Autodesk Inventor part; units mm, degrees
note: some values were not read from the file. Chosen so that the rebuilt part matches the saved one: direction of "Hole2".
(part 13 of 18)
sketch "Sketch13" plane through (0, 0, 0) normal (1, 0, 0) x (0, 1, 0)
  line L0 (0, -156.7871) -> (0, 91.8442)
  line L1 (0, 25) -> (0, -118.9769)
  line L2 (13.762, 0) -> (-13.762, 0)
  line L3 (-13.762, -20) -> (-13.762, 0)
  line L4 (-0.0006, -82.7054) -> (-0.0006, -41.7054)
  line L5 (6.5385, -24.5854) -> (6.5631, -24.5804)
  ellipse E0 centre (6.6616, -24.5626) end of major axis (7.4453, -24.4021) minor radius 0.0024 (6.8181, -24.5282) -> (6.5631, -24.5804) ccw
  ellipse E1 centre (6.6616, -24.5626) end of major axis (7.4453, -24.4021) minor radius 0.0024 (7.4453, -24.4021) -> (6.9932, -24.4925) ccw
  line L6 (7.4454, -24.4027) -> (7.4453, -24.4021)
  ellipse E2 centre (-6.6543, -24.5616) end of major axis (-7.438, -24.4009) minor radius 0.0024 (-6.9873, -24.4911) -> (-7.438, -24.4009) ccw
  line L7 (-5.6413, -24.7664) -> (-5.4089, -24.8139)
  line L8 (-7.4382, -24.4016) -> (-7.438, -24.4009)
  ellipse E3 centre (6.1292, -24.7063) end of major axis (6.8873, -24.4508) minor radius 0.0023 (6.1976, -24.6808) -> (6.0462, -24.7319) ccw
  ellipse E4 centre (6.1292, -24.7063) end of major axis (6.8873, -24.4508) minor radius 0.0023 (6.3158, -24.6411) -> (6.2034, -24.6789) ccw
  ellipse E5 centre (6.1292, -24.7063) end of major axis (6.8873, -24.4508) minor radius 0.0023 (6.8873, -24.4508) -> (6.7158, -24.5071) ccw
  line L9 (6.89, -24.4589) -> (6.8873, -24.4508)
  line L10 (4.3307, -24.5603) -> (2.6776, -19.6543)
  ellipse E6 centre (8.7715, -25.6199) end of major axis (7.994, -25.8086) minor radius 0.1369 (8.4767, -25.559) -> (8.4597, -25.5643) ccw
  line L11 (8.1889, -25.6311) -> (8.3795, -25.5808)
  ellipse E7 centre (9.0039, -26.5774) end of major axis (8.518, -26.6953) minor radius 0.0856 (8.8835, -26.5204) -> (8.737, -26.7137) ccw
  ellipse E8 centre (-9.6869, -24.5347) end of major axis (-10.4866, -24.5548) minor radius 0.1339 (-10.0381, -24.4229) -> (-10.4866, -24.5548) ccw
  line L12 (-9.714, -24.4015) -> (-8.1405, -24.3541)
  line L13 (-8.1405, -24.3541) -> (-8.1355, -24.5515)
  ellipse E9 centre (-9.6374, -26.5059) end of major axis (-10.4371, -26.526) minor radius 0.1339 (-9.3653, -26.3732) -> (-9.6644, -26.3726) ccw
  line L14 (-8.1405, -24.3541) -> (-8.1504, -23.9607)
  line L15 (-8.1673, -23.2858) -> (-8.1916, -22.3201)
  ellipse E10 centre (-10.031, -10.8352) end of major axis (-12.1204, -10.8877) minor radius 0.3499 (-10.885, -10.5366) -> (-11.1398, -10.5656) ccw
  ellipse E11 centre (-10.0087, -11.7222) end of major axis (-12.0981, -11.7747) minor radius 0.3499 (-10.8714, -11.4245) -> (-11.107, -11.4513) ccw
  ellipse E12 centre (-10.0087, -11.7222) end of major axis (-11.5083, -11.7599) minor radius 0.2511 (-9.2151, -11.4897) -> (-11.4645, -11.818) ccw
  ellipse E13 centre (-9.6374, -26.5059) end of major axis (-10.1372, -26.5184) minor radius 0.0837 (-9.7111, -26.4249) -> (-9.8858, -26.5846) ccw
  ellipse E14 centre (-7.235, -24.4816) end of major axis (-8.033, -24.4244) minor radius 0.0023 (-7.3492, -24.4711) -> (-8.033, -24.4244) ccw
  line L16 (-7.3492, -24.4711) -> (-7.2905, -24.4753)
  line L17 (-7.0539, -24.4922) -> (-5.7945, -24.5819)
  line L18 (-5.7945, -24.5819) -> (-5.8098, -24.7955)
  line L19 (-8.0339, -24.4376) -> (-8.033, -24.4244)
  line L20 (-5.7945, -24.5819) -> (-5.6751, -22.9169)
  line L21 (6.125, -24.1477) -> (6.1927, -24.4898)
  line L22 (5.1567, -24.9711) -> (6.63, -24.6998)
  ellipse E15 centre (6.6974, -24.5888) end of major axis (7.4822, -24.4335) minor radius 0.0964 (6.63, -24.6998) -> (7.3393, -24.4071) ccw
  line L23 (7.3393, -24.4071) -> (6.8175, -24.416)
  line L24 (7.4837, -24.4412) -> (7.4822, -24.4335)
  line L25 (8.6391, -24.2658) -> (8.65, -24.3696)
  line L26 (8.1334, -24.5735) -> (9.0091, -24.4769)
  ellipse E16 centre (9.1156, -24.4999) end of major axis (9.9112, -24.4166) minor radius 0.0342 (9.8759, -24.4103) -> (9.0091, -24.4769) ccw
  ellipse E17 centre (7.6703, -10.688) end of major axis (9.7489, -10.4705) minor radius 0.0893 (9.6066, -10.4531) -> (9.1054, -10.4731) ccw
  ellipse E18 centre (7.7639, -11.5823) end of major axis (9.8425, -11.3648) minor radius 0.0893 (9.6975, -11.3474) -> (9.6301, -11.3478) ccw
  ellipse E19 centre (9.3235, -26.4872) end of major axis (8.8262, -26.5392) minor radius 0.0214 (8.9471, -26.5125) -> (8.8496, -26.5302) ccw
  ellipse E20 centre (9.3235, -26.4872) end of major axis (9.8208, -26.4352) minor radius 0.0214 (9.7809, -26.431) -> (9.5114, -26.4477) ccw
  ellipse E21 centre (-3.2965, -25.8221) end of major axis (-2.5903, -25.9681) minor radius 0.4312 (-4.0047, -25.7714) -> (-3.988, -25.8345) ccw
  line L27 (-7.6925, -23.8764) -> (-7.7511, -24.4362)
  ellipse E22 centre (-9.1083, -24.4985) end of major axis (-8.3127, -24.5819) minor radius 0.0342 (-9.1389, -24.461) -> (-9.8417, -24.4085) ccw
  line L28 (-9.1389, -24.461) -> (-8.1258, -24.5652)
  line L29 (-7.5559, -24.4522) -> (-7.4967, -23.887)
  ellipse E23 centre (-7.6609, -10.6868) end of major axis (-9.7396, -10.469) minor radius 0.0893 (-9.096, -10.4717) -> (-9.5972, -10.4516) ccw
  ellipse E24 centre (-7.7547, -11.5811) end of major axis (-9.8333, -11.3633) minor radius 0.0893 (-9.6209, -11.3463) -> (-9.6883, -11.3459) ccw
  ellipse E25 centre (-7.7547, -11.5811) end of major axis (-9.2465, -11.4248) minor radius 0.0641 (-9.2062, -11.4144) -> (-9.2096, -11.4432) ccw
  ellipse E26 centre (-9.3166, -26.4858) end of major axis (-8.8193, -26.5379) minor radius 0.0214 (-8.8502, -26.542) -> (-8.9401, -26.5111) ccw
  ellipse E27 centre (-9.3166, -26.4858) end of major axis (-9.8139, -26.4337) minor radius 0.0214 (-9.5044, -26.4462) -> (-9.7826, -26.4445) ccw
  line L30 (-4.8207, -21.8442) -> (-5.4206, -24.8731)
  line L31 (-7.1249, -24.4201) -> (-7.2028, -24.4133)
  ellipse E28 centre (-6.6902, -24.5878) end of major axis (-7.4749, -24.4323) minor radius 0.0964 (-7.2028, -24.4133) -> (-6.8152, -24.6604) ccw
  line L32 (-6.8152, -24.6604) -> (-5.2896, -24.9888)
  line L33 (-5.2896, -24.9888) -> (-5.2988, -25.0352)
  line L34 (-7.4764, -24.4401) -> (-7.4749, -24.4323)
  line L35 (-5.345, -24.9535) -> (-5.2896, -24.9888)
  line L36 (-5.2896, -24.9888) -> (-4.6702, -21.8618)
  line L37 (6.9927, -24.4983) -> (7.1608, -24.4862)
  ellipse E29 centre (7.2423, -24.4827) end of major axis (8.0402, -24.4257) minor radius 0.0023 (8.0402, -24.4257) -> (7.1608, -24.4862) ccw
  line L38 (8.0412, -24.4388) -> (8.0402, -24.4257)
  line L39 (5.3972, -21.7895) -> (5.3965, -21.7786)
  line L40 (9.2707, -24.1962) -> (9.2658, -24.3887)
  line L41 (8.0528, -24.399) -> (9.5835, -24.4008)
  ellipse E30 centre (9.6941, -24.5362) end of major axis (10.4939, -24.5564) minor radius 0.1339 (10.4939, -24.5564) -> (9.5835, -24.4008) ccw
  ellipse E31 centre (10.0403, -10.8367) end of major axis (7.951, -10.7839) minor radius 0.3499 (11.1492, -10.5673) -> (10.8944, -10.5383) ccw
  ellipse E32 centre (10.0179, -11.7237) end of major axis (7.9286, -11.6709) minor radius 0.3499 (11.1162, -11.453) -> (10.8807, -11.4262) ccw
  ellipse E33 centre (10.0179, -11.7237) end of major axis (11.5174, -11.7616) minor radius 0.2511 (11.4536, -11.8315) -> (9.2243, -11.4911) ccw
  ellipse E34 centre (9.6692, -25.5218) end of major axis (8.8695, -25.5015) minor radius 0.1339 (9.5586, -25.3864) -> (9.5386, -25.3864) ccw
  ellipse E35 centre (9.6443, -26.5073) end of major axis (9.1445, -26.4947) minor radius 0.0837 (9.8928, -26.5861) -> (9.9159, -26.5843) ccw
  ellipse E36 centre (9.6443, -26.5073) end of major axis (10.1441, -26.52) minor radius 0.0837 (9.9692, -26.4517) -> (9.718, -26.4263) ccw
  line L42 (-8.2953, -25.5869) -> (-8.181, -25.6135)
  ellipse E37 centre (-8.7644, -25.6186) end of major axis (-9.5418, -25.4298) minor radius 0.1369 (-8.4526, -25.563) -> (-8.4712, -25.5572) ccw
  ellipse E38 centre (-8.9969, -26.576) end of major axis (-8.5111, -26.694) minor radius 0.0856 (-8.73, -26.7124) -> (-8.8766, -26.5191) ccw
  ellipse E39 centre (-6.122, -24.7054) end of major axis (-6.8801, -24.4498) minor radius 0.0023 (-6.7099, -24.5056) -> (-6.8801, -24.4498) ccw
  line L43 (-4.9025, -25.6565) -> (-5.0575, -26.1165)
  line L44 (-6.8828, -24.4579) -> (-6.8801, -24.4498)
  line L45 (-3.9973, -22.9715) -> (-2.7633, -19.311)
  line L46 (-4.8183, -25.9908) -> (-5.0575, -26.1165)
  line L47 (-5.0575, -26.1165) -> (-5.0809, -26.1089)
  line L48 (-5.3806, -26.0077) -> (-5.0575, -26.1165)
  line L49 (6.358, -24.6267) -> (6.5138, -24.5921)
  ellipse E40 centre (6.5935, -24.5771) end of major axis (7.3746, -24.4044) minor radius 0.0026 (6.6422, -24.5638) -> (6.5138, -24.5921) ccw
  ellipse E41 centre (6.5935, -24.5771) end of major axis (7.3746, -24.4044) minor radius 0.0026 (6.7584, -24.5381) -> (6.6452, -24.5631) ccw
  ellipse E42 centre (6.5935, -24.5771) end of major axis (7.3746, -24.4044) minor radius 0.0026 (7.3746, -24.4044) -> (6.9573, -24.4944) ccw
  line L50 (7.3751, -24.4065) -> (7.3746, -24.4044)
  ellipse E43 centre (9.3228, -26.6242) end of major axis (10.1179, -26.5359) minor radius 0.2631 (8.6364, -26.8259) -> (8.7826, -26.8719) ccw
  ellipse E44 centre (9.3228, -26.6242) end of major axis (10.1179, -26.5359) minor radius 0.2631 (9.8842, -26.7562) -> (10.0487, -26.6608) ccw
  ellipse E45 centre (-9.3159, -26.6228) end of major axis (-10.111, -26.5344) minor radius 0.2631 (-9.8452, -26.3729) -> (-9.9962, -26.4182) ccw
  ellipse E46 centre (-9.3159, -26.6228) end of major axis (-10.111, -26.5344) minor radius 0.2631 (-10.0265, -26.4334) -> (-10.0354, -26.4386) ccw
  ellipse E47 centre (-9.3159, -26.6228) end of major axis (-10.111, -26.5344) minor radius 0.2631 (-10.102, -26.5857) -> (-9.8773, -26.7547) ccw
  ellipse E48 centre (-9.3159, -26.6228) end of major axis (-8.5208, -26.7113) minor radius 0.2631 (-8.7757, -26.8706) -> (-8.6295, -26.8246) ccw
  line L51 (4.4092, -25.3666) -> (4.5281, -25.3204)
  ellipse E49 centre (5.9388, -24.7753) end of major axis (6.6846, -24.4859) minor radius 0.0025 (6.0605, -24.7254) -> (6.044, -24.7318) ccw
  ellipse E50 centre (5.9388, -24.7753) end of major axis (6.6846, -24.4859) minor radius 0.0025 (6.1548, -24.6889) -> (6.1064, -24.7077) ccw
  ellipse E51 centre (5.9388, -24.7753) end of major axis (6.6846, -24.4859) minor radius 0.0025 (6.6846, -24.4859) -> (6.6131, -24.5125) ccw
  line L52 (4.7709, -26.2989) -> (4.4092, -25.3666)
  ellipse E52 centre (6.6622, -26.6398) end of major axis (5.9164, -26.9292) minor radius 0.0025 (6.3614, -26.7541) -> (6.3717, -26.755) ccw
  line L53 (5.9164, -26.9292) -> (5.5547, -25.9969)
  line L54 (6.6905, -24.5011) -> (6.6846, -24.4859)
  line L55 (4.4092, -25.3666) -> (2.4772, -20.3874)
  line L56 (5.5556, -25.9992) -> (4.7709, -26.2989)
  line L57 (4.7709, -26.2989) -> (4.4206, -26.1135)
  ellipse E53 centre (4.7483, -25.9883) end of major axis (3.8736, -25.6036) minor radius 0.2554 (3.8766, -25.6768) -> (4.4206, -26.1135) ccw
  line L58 (3.8766, -25.6768) -> (2.3761, -21.8095)
  ellipse E54 centre (6.3005, -25.7075) end of major axis (5.5547, -25.9969) minor radius 0.0025 (5.7011, -25.9386) -> (5.5547, -25.9969) ccw
  line L59 (4.7709, -26.2989) -> (5.6964, -25.9395)
  ellipse E55 centre (6.6622, -26.6398) end of major axis (6.1961, -26.8207) minor radius 0.0015 (6.3638, -26.7544) -> (6.3692, -26.7548) ccw
  ellipse E56 centre (8.6322, -25.6643) end of major axis (7.8635, -25.8859) minor radius 0.1461 (8.4225, -25.5765) -> (8.1906, -25.6627) ccw
  line L60 (8.1897, -25.6455) -> (8.4148, -25.5772)
  ellipse E57 centre (8.9045, -26.609) end of major axis (8.4241, -26.7475) minor radius 0.0913 (8.8813, -26.5207) -> (8.7454, -26.7428) ccw
  ellipse E58 centre (8.9045, -26.609) end of major axis (8.1358, -26.8306) minor radius 0.1461 (8.5773, -26.5625) -> (8.6364, -26.8259) ccw
  line L61 (8.1358, -26.8306) -> (8.0248, -26.4453)
  line L62 (0.6093, -23.6195) -> (0.581, -23.1628)
  line L63 (-4.4761, -26.0441) -> (-4.3988, -26.1802)
  line L64 (-4.3988, -26.1802) -> (-3.922, -26.0734)
  ellipse E59 centre (-2.6442, -26.5919) end of major axis (-3.4175, -26.7969) minor radius 0.1421 (-3.4175, -26.7969) -> (-2.9999, -26.8134) ccw
  line L65 (-3.4175, -26.7969) -> (-3.5926, -26.1367)
  line L66 (-9.1967, -24.375) -> (-9.2054, -24.2017)
  line L67 (-8.4493, -24.2774) -> (-8.4463, -24.3379)
  ellipse E60 centre (-9.7984, -24.5479) end of major axis (-10.5974, -24.5882) minor radius 0.143 (-10.0811, -24.4278) -> (-10.5974, -24.5882) ccw
  line L68 (-9.8008, -24.4048) -> (-8.2279, -24.3271)
  line L69 (-8.2279, -24.3271) -> (-8.2264, -24.3567)
  ellipse E61 centre (-9.6992, -26.5132) end of major axis (-10.4982, -26.5535) minor radius 0.143 (-10.019, -26.3976) -> (-10.0418, -26.6592) ccw
  ellipse E62 centre (-9.6992, -26.5132) end of major axis (-10.4982, -26.5535) minor radius 0.143 (-9.4284, -26.3652) -> (-9.7016, -26.3701) ccw
  line L70 (-10.4982, -26.5535) -> (-10.5974, -24.5882)
  line L71 (-8.2279, -24.3271) -> (-8.2297, -24.2921)
  line L72 (-8.2813, -23.2694) -> (-8.3227, -22.4484)
  line L73 (-9.4151, -24.3858) -> (-9.4257, -24.1752)
  ellipse E63 centre (-10.4879, -10.8891) end of major axis (-12.5753, -10.9944) minor radius 0.3735 (-11.1398, -10.5656) -> (-12.5753, -10.9944) ccw
  ellipse E64 centre (-10.4433, -11.7735) end of major axis (-12.5306, -11.8788) minor radius 0.3735 (-11.107, -11.4513) -> (-12.078, -12.0859) ccw
  line L74 (-12.5753, -10.9944) -> (-12.5306, -11.8788)
  ellipse E65 centre (-10.4433, -11.7735) end of major axis (-11.9414, -11.8491) minor radius 0.2681 (-9.223, -11.5581) -> (-11.7856, -11.9582) ccw
  ellipse E66 centre (-9.6992, -26.5132) end of major axis (-10.1986, -26.5384) minor radius 0.0894 (-9.7147, -26.4245) -> (-9.8848, -26.6053) ccw
  line L75 (-6.5614, -24.4561) -> (-6.5388, -24.026)
  line L76 (-5.9229, -22.8891) -> (-5.9331, -23.0834)
  line L77 (-5.9865, -24.0968) -> (-6.0099, -24.5422)
  ellipse E67 centre (-7.32, -24.4764) end of major axis (-8.1189, -24.4343) minor radius 0.0026 (-7.411, -24.469) -> (-8.1189, -24.4343) ccw
  line L78 (-7.411, -24.469) -> (-5.8485, -24.5507)
  line L79 (-5.8485, -24.5507) -> (-5.85, -24.5779)
  ellipse E68 centre (-7.4252, -26.4736) end of major axis (-8.2241, -26.4315) minor radius 0.0026 (-7.7623, -26.4535) -> (-7.7529, -26.4587) ccw
  line L80 (-8.2241, -26.4315) -> (-8.1189, -24.4343)
  line L81 (-5.8485, -24.5507) -> (-5.7621, -22.9093)
  line L82 (-6.7227, -24.4458) -> (-6.7103, -24.2105)
  ellipse E69 centre (-7.4252, -26.4736) end of major axis (-7.9245, -26.4473) minor radius 0.0016 (-7.7601, -26.4548) -> (-7.7552, -26.4574) ccw
  line L83 (5.1995, -24.4697) -> (4.6479, -21.866)
  ellipse E70 centre (6.6428, -24.6191) end of major axis (8.0124, -24.3289) minor radius 0.2113 (6.0952, -24.5344) -> (6.0713, -24.5411) ccw
  line L84 (6.018, -24.1704) -> (6.0952, -24.5344)
  line L85 (5.0673, -25.0571) -> (5.1639, -25.008)
  line L86 (6.0952, -24.5344) -> (6.1717, -24.4955)
  line L87 (5.0673, -25.0571) -> (6.6072, -24.7497)
  ellipse E71 centre (6.6428, -24.6191) end of major axis (7.4254, -24.4532) minor radius 0.1207 (6.6072, -24.7497) -> (7.2643, -24.4155) ccw
  line L88 (7.2643, -24.4155) -> (6.3482, -24.4166)
  line L89 (5.2722, -26.0242) -> (5.0673, -25.0571)
  ellipse E72 centre (7.0526, -26.5532) end of major axis (6.2699, -26.719) minor radius 0.1207 (6.3614, -26.7541) -> (7.7692, -26.4547) ccw
  line L90 (7.4271, -24.4611) -> (7.4254, -24.4532)
  line L91 (5.0673, -25.0571) -> (4.3964, -21.8906)
  line L92 (5.2722, -26.0242) -> (4.9504, -25.7665)
  ellipse E73 centre (5.2676, -25.6052) end of major axis (4.474, -25.0398) minor radius 0.32 (4.4579, -25.1606) -> (4.9504, -25.7665) ccw
  line L93 (4.4579, -25.1606) -> (3.1313, -18.8997)
  line L94 (5.2722, -26.0242) -> (6.8121, -25.7167)
  line L95 (7.68, -24.4437) -> (7.6167, -23.8821)
  line L96 (8.5539, -24.2743) -> (8.5644, -24.367)
  line L97 (8.1344, -24.5919) -> (9.0035, -24.4922)
  ellipse E74 centre (9.0797, -24.5007) end of major axis (9.8747, -24.4111) minor radius 0.017 (9.862, -24.4095) -> (9.0035, -24.4922) ccw
  ellipse E75 centre (9.3036, -26.4876) end of major axis (8.5087, -26.5772) minor radius 0.017 (10.0259, -26.3991) -> (8.5773, -26.5625) ccw
  line L98 (7.4155, -24.403) -> (7.3584, -23.8958)
  ellipse E76 centre (7.5234, -10.6913) end of major axis (9.6002, -10.4572) minor radius 0.0445 (9.532, -10.4536) -> (9.1067, -10.4839) ccw
  ellipse E77 centre (7.6241, -11.5854) end of major axis (9.701, -11.3513) minor radius 0.0445 (9.6301, -11.3478) -> (9.211, -11.3777) ccw
  ellipse E78 centre (9.1917, -25.4942) end of major axis (8.3967, -25.5838) minor radius 0.017 (9.1154, -25.4857) -> (8.4225, -25.5765) ccw
  line L99 (8.1869, -25.5922) -> (9.1154, -25.4857)
  ellipse E79 centre (9.3036, -26.4876) end of major axis (8.8068, -26.5436) minor radius 0.0106 (9.7782, -26.431) -> (8.8144, -26.5409) ccw
  line L100 (1.5831, -23.6196) -> (1.6328, -23.1629)
  line L101 (3.6705, -25.5155) -> (2.5198, -25.5091)
  line L102 (2.6783, -26.0894) -> (3.9903, -26.0967)
  line L103 (3.9903, -26.0967) -> (4.0965, -25.9234)
  ellipse E80 centre (3.4228, -25.9197) end of major axis (4.1345, -25.7355) minor radius 0.3717 (3.8186, -25.5271) -> (3.6705, -25.5155) ccw
  ellipse E81 centre (3.4228, -25.9197) end of major axis (4.1345, -25.7355) minor radius 0.3717 (4.0965, -25.9234) -> (4.1011, -25.9156) ccw
  ellipse E82 centre (2.2762, -26.6346) end of major axis (3.0715, -26.7212) minor radius 0.2736 (2.891, -26.8683) -> (3.0068, -26.8139) ccw
  line L104 (-1.412, -23.6194) -> (-1.4616, -23.1626)
  ellipse E83 centre (-3.272, -25.9438) end of major axis (-2.5643, -26.037) minor radius 0.4004 (-3.4392, -25.5374) -> (-3.9617, -25.9767) ccw
  line L105 (-3.9803, -25.9052) -> (-3.9956, -25.7647)
  line L106 (-2.5084, -25.4929) -> (-3.4392, -25.5374)
  line L107 (-3.9617, -25.9767) -> (-3.8901, -26.1509)
  line L108 (-3.8901, -26.1509) -> (-2.6723, -26.0928)
  ellipse E84 centre (-2.2693, -26.6343) end of major axis (-3.0646, -26.7208) minor radius 0.2736 (-2.9999, -26.8134) -> (-2.8842, -26.8678) ccw
  ellipse E85 centre (-9.0725, -24.4993) end of major axis (-9.8674, -24.4096) minor radius 0.017 (-9.0782, -24.4815) -> (-9.8547, -24.408) ccw
  line L109 (-9.0782, -24.4815) -> (-8.1271, -24.5886)
  ellipse E86 centre (-9.2967, -26.4862) end of major axis (-10.0916, -26.3965) minor radius 0.017 (-8.5704, -26.5612) -> (-10.019, -26.3976) ccw
  line L110 (-7.4846, -24.4039) -> (-7.4267, -23.8907)
  ellipse E87 centre (-7.514, -10.6901) end of major axis (-9.5908, -10.4557) minor radius 0.0445 (-9.0973, -10.4825) -> (-9.5908, -10.4557) ccw
  ellipse E88 centre (-7.6149, -11.5842) end of major axis (-9.6917, -11.3499) minor radius 0.0445 (-9.2018, -11.3763) -> (-9.6209, -11.3463) ccw
  line L111 (-9.1903, -25.475) -> (-8.1797, -25.5888)
  ellipse E89 centre (-9.1846, -25.4928) end of major axis (-8.3896, -25.5825) minor radius 0.017 (-8.4154, -25.5752) -> (-9.1903, -25.475) ccw
  ellipse E90 centre (-9.2967, -26.4862) end of major axis (-9.7935, -26.4302) minor radius 0.0106 (-8.8531, -26.5411) -> (-9.7455, -26.4402) ccw
  line L112 (-6.1774, -24.4806) -> (-7.1621, -24.4178)
  ellipse E91 centre (-6.6355, -24.618) end of major axis (-7.4181, -24.4521) minor radius 0.1207 (-7.1621, -24.4178) -> (-6.7402, -24.7186) ccw
  line L113 (-6.7402, -24.7186) -> (-5.2126, -25.0673)
  line L114 (-5.2126, -25.0673) -> (-5.4176, -26.0343)
  ellipse E92 centre (-7.0456, -26.5521) end of major axis (-7.8282, -26.3862) minor radius 0.1207 (-7.7623, -26.4535) -> (-6.3545, -26.7532) ccw
  line L115 (-7.4198, -24.46) -> (-7.4181, -24.4521)
  line L116 (-5.2454, -25.0439) -> (-5.2126, -25.0673)
  line L117 (-5.2126, -25.0673) -> (-4.5363, -21.8775)
  ellipse E93 centre (-5.2794, -25.6433) end of major axis (-4.467, -25.0844) minor radius 0.2359 (-5.0758, -25.7885) -> (-4.4673, -25.177) ccw
  line L118 (-4.3995, -24.8682) -> (-3.1465, -18.9591)
  line L119 (-5.0758, -25.7885) -> (-5.4176, -26.0343)
  line L120 (-6.9452, -25.6857) -> (-5.4176, -26.0343)
  line L121 (5.951, -24.5474) -> (5.9283, -24.113)
  line L122 (6.7744, -24.1339) -> (6.7892, -24.416)
  line L123 (5.7058, -24.5603) -> (7.2751, -24.4776)
  ellipse E94 centre (7.3273, -24.4775) end of major axis (8.1262, -24.4355) minor radius 0.0026 (8.1262, -24.4355) -> (7.2751, -24.4776) ccw
  line L124 (5.7084, -24.6096) -> (5.7058, -24.5603)
  ellipse E95 centre (7.4321, -26.4747) end of major axis (8.231, -26.4328) minor radius 0.0026 (7.7598, -26.4599) -> (7.7692, -26.4547) ccw
  line L125 (8.231, -26.4328) -> (8.1262, -24.4355)
  line L126 (7.0349, -24.4123) -> (7.0194, -24.1165)
  line L127 (5.7058, -24.5603) -> (5.6198, -22.9213)
  ellipse E96 centre (7.4321, -26.4747) end of major axis (7.9314, -26.4485) minor radius 0.0016 (7.7622, -26.4586) -> (7.767, -26.4559) ccw
  line L128 (8.4258, -24.3627) -> (8.4297, -24.2848)
  line L129 (9.3468, -24.1871) -> (9.3365, -24.3909)
  line L130 (8.1607, -24.3545) -> (9.7257, -24.403)
  ellipse E97 centre (9.8056, -24.5494) end of major axis (10.6046, -24.5898) minor radius 0.143 (10.6046, -24.5898) -> (10.0883, -24.4293) ccw
  line L131 (8.1584, -24.3991) -> (8.1607, -24.3545)
  ellipse E98 centre (9.7061, -26.5146) end of major axis (10.5051, -26.5551) minor radius 0.143 (10.366, -26.6277) -> (10.0259, -26.3991) ccw
  line L132 (10.5051, -26.5551) -> (10.6046, -24.5898)
  line L133 (9.6015, -24.3991) -> (9.614, -24.1536)
  line L134 (8.1607, -24.3545) -> (8.1706, -24.1583)
  line L135 (8.2506, -22.5782) -> (8.2633, -22.3273)
  ellipse E99 centre (10.4972, -10.8907) end of major axis (12.5846, -10.9964) minor radius 0.3735 (12.5846, -10.9964) -> (11.1492, -10.5673) ccw
  ellipse E100 centre (10.4524, -11.775) end of major axis (12.5398, -11.8807) minor radius 0.3735 (12.1503, -12.0758) -> (11.1162, -11.453) ccw
  line L136 (12.5846, -10.9964) -> (12.5398, -11.8807)
  ellipse E101 centre (10.4524, -11.775) end of major axis (11.9505, -11.8509) minor radius 0.2681 (11.808, -11.9558) -> (9.2323, -11.5595) ccw
  ellipse E102 centre (9.7061, -26.5146) end of major axis (10.2055, -26.5399) minor radius 0.0894 (9.8917, -26.6068) -> (9.7217, -26.426) ccw
  line L137 (4.0061, -26.0709) -> (4.4911, -26.1682)
  line L138 (4.4911, -26.1682) -> (4.5004, -26.1558)
  ellipse E103 centre (2.6512, -26.5923) end of major axis (3.4244, -26.7975) minor radius 0.1421 (3.0068, -26.8139) -> (3.4244, -26.7975) ccw
  line L139 (3.4244, -26.7975) -> (3.6109, -26.0946)
  line L140 (-0.4449, -23.6194) -> (-0.4165, -23.1627)
  line L141 (-8.3909, -25.5774) -> (-8.1822, -25.6365)
  ellipse E104 centre (-8.6251, -25.663) end of major axis (-9.3938, -25.4413) minor radius 0.1461 (-8.1835, -25.6614) -> (-8.4154, -25.5752) ccw
  ellipse E105 centre (-8.8976, -26.6077) end of major axis (-8.4172, -26.7463) minor radius 0.0913 (-8.7385, -26.7415) -> (-8.8743, -26.5193) ccw
  ellipse E106 centre (-8.8976, -26.6077) end of major axis (-8.1289, -26.8294) minor radius 0.1461 (-8.6295, -26.8246) -> (-8.5704, -26.5612) ccw
  line L142 (-8.1289, -26.8294) -> (-8.0178, -26.4441)
  ellipse E107 centre (-5.9316, -24.7744) end of major axis (-6.6774, -24.4849) minor radius 0.0025 (-6.6233, -24.5049) -> (-6.6774, -24.4849) ccw
  ellipse E108 centre (-5.9316, -24.7744) end of major axis (-5.1858, -25.0639) minor radius 0.0025 (-6.6071, -24.511) -> (-6.6094, -24.5102) ccw
  line L143 (-4.5463, -25.309) -> (-4.5355, -25.3132)
  line L144 (-4.5355, -25.3132) -> (-4.8974, -26.2454)
  ellipse E109 centre (-6.6553, -26.6388) end of major axis (-5.9095, -26.9283) minor radius 0.0025 (-6.3648, -26.754) -> (-6.3545, -26.7532) ccw
  line L145 (-6.681, -24.4943) -> (-6.6774, -24.4849)
  line L146 (-5.9095, -26.9283) -> (-5.5507, -26.004)
  line L147 (-4.5355, -25.3132) -> (-4.5198, -25.2726)
  line L148 (-4.4473, -25.0858) -> (-2.533, -20.1542)
  ellipse E110 centre (-4.7476, -25.9842) end of major axis (-3.8553, -25.5915) minor radius 0.1687 (-4.5258, -26.0682) -> (-3.8567, -25.6236) ccw
  line L149 (-3.8567, -25.6236) -> (-2.2028, -21.3629)
  line L150 (-4.5258, -26.0682) -> (-4.8974, -26.2454)
  line L151 (-4.8974, -26.2454) -> (-5.5123, -26.0127)
  line L152 (-5.4759, -26.0211) -> (-4.8974, -26.2454)
  ellipse E111 centre (-6.6553, -26.6388) end of major axis (-6.1892, -26.8197) minor radius 0.0015 (-6.3623, -26.7538) -> (-6.3569, -26.7534) ccw
  line L153 (5.3916, -24.8026) -> (6.6698, -24.5584)
  ellipse E112 centre (6.7209, -24.5509) end of major axis (7.5067, -24.4009) minor radius 0.0022 (6.8696, -24.5203) -> (6.6698, -24.5584) ccw
  ellipse E113 centre (6.7209, -24.5509) end of major axis (7.5067, -24.4009) minor radius 0.0022 (7.5067, -24.4009) -> (7.0246, -24.4908) ccw
  line L154 (7.5079, -24.4074) -> (7.5067, -24.4009)
  line L155 (8.1314, -24.5347) -> (9.0714, -24.4299)
  ellipse E114 centre (7.9012, -11.7818) end of major axis (9.394, -11.6357) minor radius 0.2416 (9.3286, -11.5746) -> (9.2305, -11.5446) ccw
  ellipse E115 centre (7.9012, -11.7818) end of major axis (9.9812, -11.5782) minor radius 0.3366 (9.9078, -11.5013) -> (9.9018, -11.4984) ccw
  ellipse E116 centre (9.3431, -26.5156) end of major axis (8.8454, -26.5643) minor radius 0.0805 (8.9096, -26.5171) -> (8.8593, -26.5427) ccw
  ellipse E117 centre (9.3431, -26.5156) end of major axis (9.8407, -26.4669) minor radius 0.0805 (9.8304, -26.4527) -> (9.7163, -26.4265) ccw
  ellipse E118 centre (-6.7075, -24.5781) end of major axis (-5.922, -24.7302) minor radius 0.0868 (-6.7612, -24.4796) -> (-7.3551, -24.4041) ccw
  line L156 (-6.7612, -24.4796) -> (-6.583, -24.5123)
  line L157 (5.9989, -24.7396) -> (6.2404, -24.6679)
  ellipse E119 centre (6.2865, -24.6565) end of major axis (7.0535, -24.4291) minor radius 0.0022 (6.4331, -24.6108) -> (6.2404, -24.6679) ccw
  ellipse E120 centre (6.2865, -24.6565) end of major axis (7.0535, -24.4291) minor radius 0.0022 (6.5044, -24.5897) -> (6.5018, -24.5905) ccw
  ellipse E121 centre (6.2865, -24.6565) end of major axis (7.0535, -24.4291) minor radius 0.0022 (7.0529, -24.4291) -> (6.7995, -24.5027) ccw
  line L158 (5.0175, -26.0738) -> (4.9188, -25.7408)
  line L159 (2.9914, -18.5399) -> (2.9814, -18.5429)
  line L160 (3.7346, -21.7468) -> (2.887, -18.8882)
  line L161 (5.0288, -26.0705) -> (5.0175, -26.0738)
  line L162 (5.0175, -26.0738) -> (4.9539, -26.0338)
  line L163 (5.0175, -26.0738) -> (5.2485, -26.0052)
  line L164 (8.5899, -24.5105) -> (8.6074, -24.5066)
  ellipse E122 centre (8.682, -24.6222) end of major axis (9.4653, -24.4596) minor radius 0.1285 (8.8432, -24.4612) -> (8.6074, -24.5066) ccw
  line L165 (8.1877, -25.6082) -> (8.2509, -25.5945)
  ellipse E123 centre (9.0831, -26.555) end of major axis (8.5936, -26.6566) minor radius 0.0803 (8.8837, -26.5204) -> (8.7282, -26.6832) ccw
  ellipse E124 centre (-9.6046, -24.5259) end of major axis (-10.4046, -24.5311) minor radius 0.1258 (-9.5844, -24.4) -> (-10.4046, -24.5311) ccw
  line L166 (-9.5844, -24.4) -> (-8.8698, -24.3983)
  line L167 (-8.0317, -24.3963) -> (-8.0101, -24.3963)
  line L168 (-8.0101, -24.3963) -> (-8.0099, -24.4255)
  ellipse E125 centre (-9.5918, -26.501) end of major axis (-10.3917, -26.5062) minor radius 0.1258 (-9.3068, -26.3816) -> (-9.5715, -26.3751) ccw
  line L169 (-8.0101, -24.3963) -> (-8.0136, -23.8586)
  line L170 (-8.0201, -22.8541) -> (-8.0235, -22.3387)
  ellipse E126 centre (-9.694, -10.7991) end of major axis (-11.784, -10.8127) minor radius 0.3286 (-9.8563, -10.4725) -> (-10.885, -10.5366) ccw
  ellipse E127 centre (-9.6882, -11.6879) end of major axis (-11.7782, -11.7015) minor radius 0.3286 (-9.9328, -11.3631) -> (-10.8714, -11.4245) ccw
  ellipse E128 centre (-9.6882, -11.6879) end of major axis (-11.1882, -11.6977) minor radius 0.2359 (-9.2117, -11.4612) -> (-11.1859, -11.7106) ccw
  ellipse E129 centre (-9.5918, -26.501) end of major axis (-10.0917, -26.5042) minor radius 0.0786 (-9.7073, -26.4252) -> (-9.8868, -26.5663) ccw
  ellipse E130 centre (-7.1783, -24.4861) end of major axis (-7.9755, -24.4188) minor radius 0.0022 (-7.2621, -24.4768) -> (-7.9755, -24.4188) ccw
  line L171 (-7.9763, -24.4276) -> (-7.9755, -24.4188)
  line L172 (5.3926, -24.8024) -> (4.8437, -21.8432)
  line L173 (5.1714, -24.93) -> (5.3971, -24.8443)
  line L174 (5.1714, -24.93) -> (6.7191, -24.6513)
  ellipse E131 centre (6.7477, -24.5673) end of major axis (7.5343, -24.4214) minor radius 0.0775 (6.7191, -24.6513) -> (7.3746, -24.4045) ccw
  ellipse E132 centre (6.7477, -24.5673) end of major axis (5.9611, -24.7132) minor radius 0.0775 (7.373, -24.4046) -> (7.3678, -24.4049) ccw
  line L175 (7.3678, -24.4049) -> (7.3235, -24.4074)
  line L176 (5.1777, -24.9639) -> (5.1714, -24.93)
  line L177 (7.5405, -24.4553) -> (7.5343, -24.4214)
  line L178 (5.1714, -24.93) -> (4.9118, -23.5302)
  line L179 (7.7542, -24.4377) -> (7.6996, -23.8776)
  line L180 (8.1326, -24.5571) -> (9.0839, -24.4601)
  ellipse E133 centre (9.1469, -24.5) end of major axis (9.9431, -24.4223) minor radius 0.046 (9.8852, -24.4109) -> (9.0839, -24.4601) ccw
  line L181 (7.5002, -24.4019) -> (7.4503, -23.891)
  ellipse E134 centre (7.7987, -10.6887) end of major axis (9.8789, -10.4856) minor radius 0.1201 (9.8657, -10.474) -> (9.1048, -10.4677) ccw
  ellipse E135 centre (7.886, -11.5829) end of major axis (9.9661, -11.3799) minor radius 0.1201 (9.9421, -11.3646) -> (9.6975, -11.3474) ccw
  ellipse E136 centre (7.886, -11.5829) end of major axis (9.3789, -11.4372) minor radius 0.0862 (9.2243, -11.4911) -> (9.2153, -11.4142) ccw
  ellipse E137 centre (9.3409, -26.4873) end of major axis (9.8385, -26.4387) minor radius 0.0287 (9.7973, -26.4314) -> (9.7809, -26.431) ccw
  line L182 (-7.7083, -23.8756) -> (-7.763, -24.4352)
  ellipse E138 centre (-9.1397, -24.4987) end of major axis (-9.9359, -24.4208) minor radius 0.046 (-9.123, -24.4541) -> (-9.878, -24.4094) ccw
  line L183 (-9.123, -24.4541) -> (-8.1252, -24.5525)
  ellipse E139 centre (-7.7894, -10.6875) end of major axis (-9.8695, -10.4841) minor radius 0.1201 (-9.0954, -10.4663) -> (-9.8563, -10.4725) ccw
  ellipse E140 centre (-7.8768, -11.5817) end of major axis (-9.9569, -11.3784) minor radius 0.1201 (-9.6883, -11.3459) -> (-9.9328, -11.3631) ccw
  ellipse E141 centre (-7.8768, -11.5817) end of major axis (-9.3697, -11.4358) minor radius 0.0862 (-9.2061, -11.4128) -> (-9.2151, -11.4897) ccw
  ellipse E142 centre (-9.334, -26.4859) end of major axis (-8.8363, -26.5345) minor radius 0.0287 (-8.8553, -26.5404) -> (-8.8766, -26.5191) ccw
  ellipse E143 centre (-9.334, -26.4859) end of major axis (-9.8316, -26.4372) minor radius 0.0287 (-9.6139, -26.4347) -> (-9.8082, -26.4484) ccw
  line L184 (-4.8827, -21.837) -> (-5.4272, -24.7695)
  ellipse E144 centre (-6.7404, -24.5663) end of major axis (-7.527, -24.4203) minor radius 0.0775 (-7.3551, -24.4041) -> (-6.8165, -24.6308) ccw
  line L185 (-6.8165, -24.6308) -> (-5.338, -24.917)
  line L186 (-7.5333, -24.4541) -> (-7.527, -24.4203)
  line L187 (5.5787, -24.6206) -> (7.146, -24.4883)
  ellipse E145 centre (7.1856, -24.4871) end of major axis (7.9828, -24.42) minor radius 0.0022 (7.2677, -24.478) -> (7.146, -24.4883) ccw
  ellipse E146 centre (7.1856, -24.4871) end of major axis (7.9828, -24.42) minor radius 0.0022 (7.9828, -24.42) -> (7.2679, -24.478) ccw
  line L188 (5.5908, -24.7645) -> (5.5787, -24.6206)
  line L189 (7.9835, -24.4288) -> (7.9828, -24.42)
  line L190 (5.5787, -24.6206) -> (5.4346, -22.9109)
  line L191 (5.3422, -21.8148) -> (5.3397, -21.7853)
  line L192 (9.105, -24.2155) -> (9.1039, -24.3837)
  line L193 (7.9758, -24.412) -> (9.5451, -24.4016)
  ellipse E147 centre (9.6119, -24.5274) end of major axis (10.4118, -24.5327) minor radius 0.1258 (10.0454, -24.4245) -> (9.5451, -24.4016) ccw
  line L194 (7.9757, -24.4203) -> (7.9758, -24.412)
  line L195 (7.9758, -24.412) -> (7.9794, -23.8621)
  line L196 (7.9861, -22.8573) -> (7.9914, -22.0683)
  ellipse E148 centre (9.7033, -10.8006) end of major axis (7.6134, -10.7867) minor radius 0.3286 (10.8944, -10.5383) -> (9.8657, -10.474) ccw
  ellipse E149 centre (9.6974, -11.6894) end of major axis (7.6075, -11.6755) minor radius 0.3286 (10.8807, -11.4262) -> (9.9421, -11.3646) ccw
  ellipse E150 centre (9.6974, -11.6894) end of major axis (11.1974, -11.6994) minor radius 0.2359 (11.1795, -11.7354) -> (9.2209, -11.4626) ccw
  ellipse E151 centre (9.6053, -25.5149) end of major axis (8.8053, -25.5096) minor radius 0.1258 (9.5385, -25.3891) -> (9.2172, -25.4024) ccw
  ellipse E152 centre (9.5987, -26.5024) end of major axis (10.0987, -26.5058) minor radius 0.0786 (9.9513, -26.449) -> (9.7143, -26.4267) ccw
  line L197 (-8.192, -25.5983) -> (-8.1803, -25.6008)
  ellipse E153 centre (-9.0762, -26.5536) end of major axis (-8.5867, -26.6553) minor radius 0.0803 (-8.7213, -26.6819) -> (-8.8768, -26.519) ccw
  ellipse E154 centre (-6.2793, -24.6555) end of major axis (-7.0462, -24.428) minor radius 0.0022 (-6.7936, -24.5013) -> (-7.0457, -24.4281) ccw
  line L198 (-3.4821, -20.5418) -> (-2.9328, -18.6903)
  line L199 (-2.9735, -18.5414) -> (-2.983, -18.5386)
  ellipse E155 centre (7.9002, -22.0305) end of major axis (8.7408, -21.8264) minor radius 0.1481 (7.7792, -21.9083) -> (7.7092, -21.9272) ccw
  ellipse E156 centre (7.9002, -22.0305) end of major axis (8.7408, -21.8264) minor radius 0.1481 (7.9699, -21.8624) -> (7.9228, -21.873) ccw
  ellipse E157 centre (-9.7702, -21.2173) end of major axis (-9.3134, -21.2058) minor radius 0.0765 (-9.3901, -21.1655) -> (-9.9432, -21.1507) ccw
  ellipse E158 centre (-9.7702, -21.2173) end of major axis (-10.6349, -21.239) minor radius 0.1448 (-9.2686, -21.087) -> (-10.4771, -21.3179) ccw
  ellipse E159 centre (-9.795, -20.2317) end of major axis (-10.6597, -20.2534) minor radius 0.1448 (-9.5774, -20.0862) -> (-10.6597, -20.2534) ccw
  line L200 (-10.6597, -20.2534) -> (-10.6349, -21.239)
  ellipse E160 centre (-7.0541, -21.9571) end of major axis (-7.9169, -21.8953) minor radius 0.0025 (-6.9565, -21.9616) -> (-7.7008, -21.9124) ccw
  line L201 (-7.8875, -21.4857) -> (-7.9169, -21.8953)
  ellipse E161 centre (8.8803, -22.2512) end of major axis (8.02, -22.3412) minor radius 0.037 (9.7365, -22.1654) -> (8.0392, -22.3469) ccw
  ellipse E162 centre (8.7763, -21.2576) end of major axis (9.6366, -21.1675) minor radius 0.037 (9.6366, -21.1675) -> (8.3967, -21.2639) ccw
  line L202 (9.6366, -21.1675) -> (9.7406, -22.1612)
  line L203 (7.9301, -21.4828) -> (8.02, -22.3412)
  ellipse E163 centre (-8.8727, -22.2499) end of major axis (-9.733, -22.1597) minor radius 0.037 (-8.0124, -22.3401) -> (-9.7289, -22.1639) ccw
  ellipse E164 centre (-8.7686, -21.2562) end of major axis (-9.6288, -21.1661) minor radius 0.037 (-8.3889, -21.2626) -> (-9.6288, -21.1661) ccw
  line L204 (-7.9224, -21.4816) -> (-8.0124, -22.34)
  line L205 (-9.6288, -21.1661) -> (-9.733, -22.1597)
  ellipse E165 centre (7.0617, -21.9582) end of major axis (7.9245, -21.8965) minor radius 0.0025 (7.7084, -21.9136) -> (6.9641, -21.9626) ccw
  line L206 (7.8952, -21.4869) -> (7.9245, -21.8965)
  ellipse E166 centre (9.778, -21.2187) end of major axis (10.2348, -21.2303) minor radius 0.0765 (9.9509, -21.1522) -> (9.3979, -21.1669) ccw
  ellipse E167 centre (9.778, -21.2187) end of major axis (10.6427, -21.2406) minor radius 0.1448 (10.4848, -21.3195) -> (9.2764, -21.0884) ccw
  ellipse E168 centre (9.8029, -20.2332) end of major axis (10.6676, -20.255) minor radius 0.1448 (10.6676, -20.255) -> (9.5853, -20.0876) ccw
  line L207 (10.6676, -20.255) -> (10.6427, -21.2406)
  ellipse E169 centre (6.4648, -23.9952) end of major axis (6.0186, -24.0939) minor radius 0.0015 (6.7925, -23.9217) -> (6.0302, -24.0916) ccw
  ellipse E170 centre (6.4648, -23.9952) end of major axis (7.3094, -23.8085) minor radius 0.0028 (6.8755, -23.9019) -> (5.7844, -24.1439) ccw
  ellipse E171 centre (6.2489, -23.0188) end of major axis (7.0935, -22.832) minor radius 0.0028 (6.9755, -22.8567) -> (5.6685, -23.145) ccw
  line L208 (9.7783, -23.0095) -> (9.7899, -23.112)
  line L209 (-9.7708, -23.0081) -> (-9.7824, -23.1105)
  ellipse E172 centre (-6.4575, -23.9942) end of major axis (-6.0113, -24.0929) minor radius 0.0015 (-6.0229, -24.0907) -> (-6.7852, -23.9207) ccw
  ellipse E173 centre (-6.4575, -23.9942) end of major axis (-5.6129, -24.1811) minor radius 0.0028 (-5.9261, -24.1096) -> (-6.8681, -23.9009) ccw
  ellipse E174 centre (-6.2415, -23.0178) end of major axis (-5.3969, -23.2047) minor radius 0.0028 (-5.843, -23.1035) -> (-6.968, -22.8556) ccw
  ellipse E175 centre (6.4739, -24.121) end of major axis (6.9197, -24.0207) minor radius 0.0774 (6.6733, -24.1484) -> (6.0706, -24.175) ccw
  ellipse E176 centre (6.4739, -24.121) end of major axis (7.3178, -23.9311) minor radius 0.1465 (6.0158, -24.0948) -> (5.9289, -24.1252) ccw
  ellipse E177 centre (6.4739, -24.121) end of major axis (7.3178, -23.9311) minor radius 0.1465 (6.9279, -24.1484) -> (7.2768, -23.8993) ccw
  line L210 (7.3104, -23.8983) -> (7.3178, -23.9311)
  ellipse E178 centre (-6.4666, -24.12) end of major axis (-6.9124, -24.0196) minor radius 0.0774 (-6.0578, -24.1774) -> (-6.5794, -24.1721) ccw
  ellipse E179 centre (-6.4666, -24.12) end of major axis (-5.6227, -24.31) minor radius 0.1465 (-5.9867, -24.1012) -> (-6.0085, -24.0939) ccw
  ellipse E180 centre (-6.4666, -24.12) end of major axis (-7.3104, -23.93) minor radius 0.1465 (-7.2695, -23.8982) -> (-6.71, -24.2105) ccw
  line L211 (-7.303, -23.8972) -> (-7.3104, -23.93)
  ellipse E181 centre (5.2399, -22.9741) end of major axis (6.0464, -22.6612) minor radius 0.0027 (5.4137, -22.9039) -> (5.0655, -23.039) ccw
  ellipse E182 centre (4.8782, -22.0418) end of major axis (5.6846, -21.7289) minor radius 0.0027 (5.1866, -21.9195) -> (4.8799, -22.0383) ccw
  ellipse E183 centre (7.8177, -22.8387) end of major axis (8.6488, -22.5991) minor radius 0.158 (7.9522, -22.6393) -> (7.7494, -22.694) ccw
  ellipse E184 centre (7.8177, -22.8387) end of major axis (8.6488, -22.5991) minor radius 0.158 (8.3433, -22.5653) -> (8.0059, -22.6265) ccw
  ellipse E185 centre (-9.8759, -23.013) end of major axis (-10.3323, -23.036) minor radius 0.0817 (-9.6484, -22.931) -> (-9.7799, -23.0882) ccw
  ellipse E186 centre (-9.8759, -23.013) end of major axis (-10.7398, -23.0566) minor radius 0.1546 (-9.4057, -22.8601) -> (-9.7921, -23.1629) ccw
  ellipse E187 centre (-9.9255, -22.0303) end of major axis (-10.7894, -22.0739) minor radius 0.1546 (-9.7026, -21.8699) -> (-10.7894, -22.0739) ccw
  line L212 (-10.7894, -22.0739) -> (-10.7398, -23.0566)
  ellipse E188 centre (-7.2895, -23.8952) end of major axis (-7.7458, -23.8711) minor radius 0.0015 (-6.895, -23.9167) -> (-7.0617, -23.9084) ccw
  ellipse E189 centre (-7.2895, -23.8952) end of major axis (-8.1533, -23.8497) minor radius 0.0028 (-6.785, -23.9194) -> (-7.3031, -23.8972) ccw
  ellipse E190 centre (-7.2369, -22.8965) end of major axis (-6.3731, -22.942) minor radius 0.0028 (-6.4941, -22.9342) -> (-6.6474, -22.9255) ccw
  ellipse E191 centre (-7.2369, -22.8965) end of major axis (-8.1007, -22.8511) minor radius 0.0028 (-6.7348, -22.9207) -> (-8.1007, -22.8511) ccw
  line L213 (-8.1007, -22.8511) -> (-8.1533, -23.8497)
  ellipse E192 centre (6.2367, -22.7023) end of major axis (5.3904, -22.8816) minor radius 0.1305 (5.3904, -22.8816) -> (7.0829, -22.523) ccw
  ellipse E193 centre (6.0318, -21.7352) end of major axis (5.1855, -21.9145) minor radius 0.1305 (5.2979, -21.8205) -> (6.836, -21.6105) ccw
  line L214 (6.8883, -21.6044) -> (7.0829, -22.523)
  line L215 (5.1855, -21.9145) -> (5.3904, -22.8816)
  ellipse E194 centre (9.0462, -24.2036) end of major axis (9.5003, -24.1524) minor radius 0.0097
  ellipse E195 centre (9.0462, -24.2036) end of major axis (8.1867, -24.3005) minor radius 0.0184 (8.4296, -24.286) -> (8.2022, -24.3022) ccw
  ellipse E196 centre (8.9343, -23.2101) end of major axis (8.0747, -23.307) minor radius 0.0184 (9.7938, -23.1133) -> (8.1314, -23.294) ccw
  line L216 (9.7938, -23.1133) -> (9.9058, -24.1068)
  line L217 (8.1362, -23.8529) -> (8.1867, -24.3005)
  ellipse E197 centre (-9.0389, -24.2023) end of major axis (-9.493, -24.151) minor radius 0.0097
  ellipse E198 centre (-9.0389, -24.2023) end of major axis (-9.8985, -24.1052) minor radius 0.0184 (-8.1828, -24.2972) -> (-8.4491, -24.2823) ccw
  ellipse E199 centre (-8.9268, -23.2088) end of major axis (-9.7864, -23.1118) minor radius 0.0184 (-8.1239, -23.2927) -> (-9.7864, -23.1118) ccw
  line L218 (-9.7864, -23.1118) -> (-9.8985, -24.1052)
  ellipse E200 centre (-6.2291, -22.7014) end of major axis (-7.0753, -22.5219) minor radius 0.1305 (-7.0753, -22.5219) -> (-5.383, -22.8808) ccw
  ellipse E201 centre (-6.0241, -21.7343) end of major axis (-6.8703, -21.5549) minor radius 0.1305 (-6.8284, -21.6095) -> (-5.2091, -21.8669) ccw
  line L219 (-5.1779, -21.9137) -> (-5.383, -22.8808)
  line L220 (-6.8806, -21.6034) -> (-7.0753, -22.5219)
  ellipse E202 centre (7.2968, -23.8963) end of major axis (6.8404, -23.9202) minor radius 0.0015 (7.069, -23.9095) -> (6.9023, -23.9177) ccw
  ellipse E203 centre (7.2968, -23.8963) end of major axis (8.1606, -23.8509) minor radius 0.0028 (7.3104, -23.8983) -> (6.7923, -23.9205) ccw
  ellipse E204 centre (7.2444, -22.8976) end of major axis (8.1082, -22.8523) minor radius 0.0028 (6.6549, -22.9265) -> (6.5016, -22.9352) ccw
  ellipse E205 centre (7.2444, -22.8976) end of major axis (8.1082, -22.8523) minor radius 0.0028 (8.1082, -22.8523) -> (6.7423, -22.9217) ccw
  line L221 (8.1082, -22.8523) -> (8.1606, -23.8509)
  ellipse E206 centre (9.8834, -23.0145) end of major axis (10.3398, -23.0376) minor radius 0.0817 (9.7874, -23.0897) -> (9.6559, -22.9324) ccw
  ellipse E207 centre (9.8834, -23.0145) end of major axis (10.7473, -23.0582) minor radius 0.1546 (9.7996, -23.1644) -> (9.4132, -22.8616) ccw
  ellipse E208 centre (9.9331, -22.0318) end of major axis (10.797, -22.0756) minor radius 0.1546 (10.797, -22.0756) -> (9.7102, -21.8714) ccw
  line L222 (10.797, -22.0756) -> (10.7473, -23.0582)
  ellipse E209 centre (-7.8102, -22.8375) end of major axis (-6.9791, -23.0772) minor radius 0.158 (-7.7419, -22.6928) -> (-7.8164, -22.6716) ccw
  ellipse E210 centre (-5.2325, -22.9733) end of major axis (-4.4261, -23.2863) minor radius 0.0027 (-5.1025, -23.0209) -> (-5.2359, -22.9691) ccw
  ellipse E211 centre (-4.8706, -22.0411) end of major axis (-4.0642, -22.3541) minor radius 0.0027 (-4.9168, -22.0203) -> (-5.1052, -21.9473) ccw
  ellipse E212 centre (8.5586, -18.3649) end of major axis (9.4196, -18.2817) minor radius 0.2215 (9.1394, -18.1482) -> (9.0433, -18.1373) ccw
  ellipse E213 centre (-8.5504, -18.3636) end of major axis (-7.6894, -18.4469) minor radius 0.2215 (-9.0351, -18.1359) -> (-9.1312, -18.1468) ccw
  ellipse E214 centre (-9.6382, -19.37) end of major axis (-9.1812, -19.367) minor radius 0.0719 (-9.5006, -19.3006) -> (-9.8309, -19.306) ccw
  ellipse E215 centre (-9.6382, -19.37) end of major axis (-10.5032, -19.3756) minor radius 0.136 (-9.4942, -19.2349) -> (-10.5019, -19.368) ccw
  ellipse E216 centre (-9.6446, -18.3824) end of major axis (-10.5096, -18.3881) minor radius 0.136 (-9.0492, -18.28) -> (-10.5047, -18.3734) ccw
  ellipse E217 centre (8.7352, -20.2821) end of major axis (9.19, -20.2377) minor radius 0.0263 (9.1877, -20.2408) -> (9.1871, -20.2352) ccw
  ellipse E218 centre (8.7352, -20.2821) end of major axis (9.5961, -20.1981) minor radius 0.0497 (9.5863, -20.2068) -> (8.5502, -20.2513) ccw
  ellipse E219 centre (8.6382, -19.2885) end of major axis (9.4991, -19.2045) minor radius 0.0497 (9.4991, -19.2045) -> (8.7047, -19.2322) ccw
  line L223 (9.4991, -19.2045) -> (9.5961, -20.1981)
  ellipse E220 centre (-8.7273, -20.2808) end of major axis (-9.1821, -20.2363) minor radius 0.0263 (-9.1792, -20.2338) -> (-9.1798, -20.2394) ccw
  ellipse E221 centre (-8.7273, -20.2808) end of major axis (-9.5882, -20.1966) minor radius 0.0497 (-8.5423, -20.25) -> (-9.5784, -20.2054) ccw
  ellipse E222 centre (-8.6302, -19.2872) end of major axis (-9.4911, -19.203) minor radius 0.0497 (-8.6967, -19.2309) -> (-9.4911, -19.203) ccw
  line L224 (-9.4911, -19.203) -> (-9.5882, -20.1966)
  ellipse E223 centre (9.6462, -19.3714) end of major axis (10.1032, -19.3745) minor radius 0.0719 (9.8389, -19.3075) -> (9.5086, -19.302) ccw
  ellipse E224 centre (9.6462, -19.3714) end of major axis (10.5112, -19.3772) minor radius 0.136 (10.5099, -19.3695) -> (9.5022, -19.2364) ccw
  ellipse E225 centre (9.6528, -18.3839) end of major axis (10.5178, -18.3897) minor radius 0.136 (10.5128, -18.375) -> (9.0573, -18.2814) ccw
  ellipse E226 centre (0.0096, 53.5061) end of major axis (0.0755, 54.2464) minor radius 0.1949 (0.2146, 53.7278) -> (-0.1955, 53.2845) ccw
  line L225 (-0.1956, 51.2748) -> (-0.1955, 53.2845)
  line L226 (0.2144, 51.7176) -> (0.2146, 53.7278)
  ellipse E227 centre (2.1439, 53.5064) end of major axis (2.2871, 54.2605) minor radius 0.1955 (2.371, 53.7068) -> (2.0961, 54.0361) ccw
  line L227 (-0.3412, 31.7407) -> (-0.257, 32.5448)
  line L228 (2.2095, 52.1647) -> (2.371, 53.7068)
  ellipse E228 centre (-2.1248, 53.5067) end of major axis (-2.1408, 54.2741) minor radius 0.1955 (-2.0989, 54.2575) -> (-2.3055, 53.2638) ccw
  line L229 (-2.2004, 52.259) -> (-2.3055, 53.2638)
  line L230 (0.357, 31.7407) -> (0.2729, 32.5448)
  ellipse E229 centre (0.0094, 51.4962) end of major axis (0.0756, 52.2332) minor radius 0.1948 (0.2144, 51.7176) -> (-0.1956, 51.2748) ccw
  line L231 (-0.1969, 34.7396) -> (-0.1956, 51.2748)
  line L232 (0.2131, 34.7395) -> (0.2144, 51.7176)
  ellipse E230 centre (2.1749, 51.4959) end of major axis (2.3272, 52.2482) minor radius 0.1955 (2.4044, 51.6935) -> (2.1059, 51.9606) ccw
  line L233 (-1.1612, 24.7267) -> (-0.3412, 31.7409)
  line L234 (0.2249, 33.0517) -> (2.4044, 51.6935)
  line L235 (-0.1976, 24.7248) -> (-0.1971, 31.2292)
  line L236 (0.2124, 24.7247) -> (0.2129, 31.2292)
  ellipse E231 centre (-2.1561, 51.4962) end of major axis (-2.1814, 52.2634) minor radius 0.1955 (-2.116, 52.2232) -> (-2.3338, 51.2511) ccw
  line L237 (-0.2089, 33.0517) -> (-2.3338, 51.2511)
  line L238 (1.1759, 24.7265) -> (0.357, 31.7408)
  ellipse E232 centre (0.0097, 55.5342) end of major axis (0.0736, 56.2991) minor radius 0.1955 (0.2147, 55.7571) -> (-0.1953, 55.3114) ccw
  line L239 (-0.1953, 55.2903) -> (-0.1953, 55.3114)
  line L240 (0.2147, 55.7341) -> (0.2147, 55.7571)
  ellipse E233 centre (0.0097, 55.5122) end of major axis (0.0755, 56.2552) minor radius 0.1949 (0.2147, 55.7341) -> (-0.1953, 55.2903) ccw
  line L241 (-0.1955, 53.2845) -> (-0.1953, 55.2903)
  line L242 (0.2146, 53.7278) -> (0.2147, 55.7341)
  ellipse E234 centre (2.1278, 55.5129) end of major axis (2.2636, 56.2683) minor radius 0.1955 (2.3529, 55.7155) -> (1.9026, 55.3103) ccw
  ellipse E235 centre (-0.7937, 24.7162) end of major axis (-0.5896, 24.6969) minor radius 0 (-0.5896, 24.6969) -> (-0.8355, 24.7202) ccw
  line L243 (-0.2571, 32.5439) -> (-0.2089, 33.0518)
  line L244 (0.2133, 37.5027) -> (1.9026, 55.3103)
  line L245 (-0.5896, 24.6969) -> (-0.1973, 28.8323)
  line L246 (2.2116, 54.2264) -> (2.3529, 55.7155)
  ellipse E236 centre (-2.1083, 55.5132) end of major axis (-2.1169, 56.2807) minor radius 0.1955 (-1.9253, 55.7544) -> (-2.2914, 55.272) ccw
  ellipse E237 centre (0.8084, 24.7161) end of major axis (0.6043, 24.6968) minor radius 0 (0.8502, 24.7201) -> (0.6043, 24.6968) ccw
  line L247 (0.6043, 24.6968) -> (0.2127, 28.8322)
  line L248 (-2.194, 54.2433) -> (-2.2914, 55.272)
  line L249 (0.273, 32.5439) -> (0.2249, 33.0518)
  line L250 (-0.1967, 37.5027) -> (-1.9253, 55.7544)
  line L251 (-9.0479, -18.0189) -> (-9.0222, -18.0039)
  line L252 (-9.1063, -17.8989) -> (-9.0992, -17.9004)
  line L253 (-9.1327, -17.9142) -> (-9.1063, -17.8989)
  line L254 (-9.1063, -17.8989) -> (-9.1032, -17.869)
  line L255 (-10.7112, -17.8662) -> (-10.6939, -17.867)
  line L256 (-10.6939, -17.867) -> (-10.6465, -17.8472)
  line L257 (-10.543, -17.8039) -> (-10.5099, -17.79)
  line L258 (-10.3387, -17.7184) -> (-10.3146, -17.7083)
  line L259 (-10.5078, -17.6992) -> (-10.3146, -17.7083)
  line L260 (-10.5895, -17.7334) -> (-10.5078, -17.6992)
  line L261 (-10.3146, -17.7083) -> (-10.3146, -17.707)
  line L262 (-10.5078, -17.6992) -> (-10.5092, -17.6427)
  line L263 (-10.5555, -15.7989) -> (-10.5555, -15.7986)
  line L264 (-10.6081, -13.7049) -> (-10.6087, -13.6801)
  line L265 (-9.944, -17.6474) -> (-9.9811, -17.6629)
  line L266 (-9.9443, -17.6343) -> (-9.944, -17.6474)
  line L267 (-9.944, -17.6474) -> (-9.8266, -17.6529)
  line L268 (-9.6767, -17.6599) -> (-9.1925, -17.6825)
  line L269 (9.2395, -17.7312) -> (9.2664, -17.729)
  line L270 (9.5099, -17.7086) -> (9.5186, -17.7078)
  line L271 (9.7738, -17.6445) -> (9.7991, -17.6517)
  line L272 (9.7145, -17.6495) -> (9.7738, -17.6445)
  line L273 (9.7738, -17.6445) -> (9.7742, -17.6259)
  line L274 (10.1944, -17.6017) -> (10.192, -17.6952)
  line L275 (10.3682, -17.6804) -> (10.192, -17.6952)
  line L276 (10.4698, -13.6599) -> (10.4694, -13.6781)
  line L277 (10.4163, -15.7798) -> (10.4157, -15.801)
  line L278 (10.3699, -17.6133) -> (10.3682, -17.6804)
  line L279 (10.192, -17.6952) -> (10.3159, -17.7303)
  line L280 (10.5983, -17.8103) -> (10.6113, -17.814)
  line L281 (10.3682, -17.6804) -> (10.5267, -17.7253)
  line L282 (10.6767, -17.9003) -> (10.6582, -17.8951)
  line L283 (9.1349, -17.7541) -> (9.1478, -17.7564)
  line L284 (-10.646, -17.9728) -> (-10.8715, -17.9652)
  line L285 (-10.9595, -18.0036) -> (-10.8715, -17.9652)
  line L286 (-10.6439, -18.0143) -> (-10.9595, -18.0036)
  line L287 (-10.9595, -18.0036) -> (-10.9618, -17.9567)
  line L288 (-11.1692, -17.9117) -> (-10.9788, -17.9182)
  line L289 (-11.172, -17.8568) -> (-11.1692, -17.9117)
  line L290 (-10.9788, -17.9182) -> (-10.5725, -17.7407)
  line L291 (-10.7629, -17.7343) -> (-10.5725, -17.7407)
  line L292 (-11.1692, -17.9117) -> (-10.7629, -17.7343)